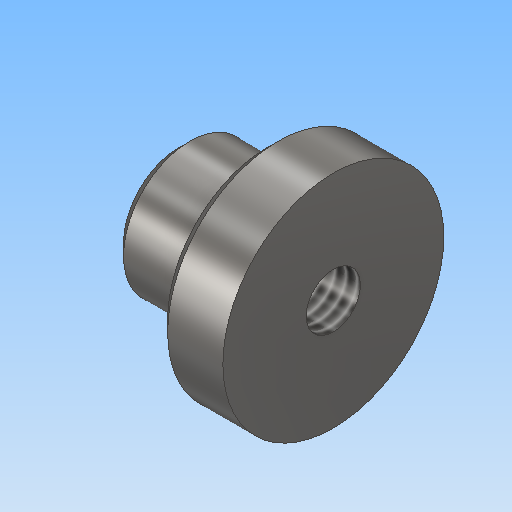
# Autodesk Inventor part: Top_Shaft 1
Saved by Autodesk Inventor 2018.1 (Build 221171000, 171)
## iProperties
Created: 2019-03-18
Part Number: Top_Shaft 1
Material: Stainless Steel
Document SubType Name: Modeling
Designer: James
Density: 8 g/cm^3
Appearance: Semi-Polished
Mass: 2.47594 g
Surface Area: 3.55126 cm^2
Volume: 0.309493 cm^3
Author: James
Autodesk Inventor part; units mm, degrees
ref_plane "YZ Plane" through (0, 0, 0) normal (1, 0, 0) x (0, 1, 0)
ref_plane "XZ Plane" through (0, 0, 0) normal (0, 1, 0) x (-1, 0, 0)
ref_plane "XY Plane" through (0, 0, 0) normal (0, 0, 1) x (1, 0, 0)
sketch "Sketch1" plane through (0, 0, 0) normal (0, 0, 1) x (1, 0, 0)
  line L0 (0, 0) -> (4, 0)
  line L1 (4, 0) -> (4, 3)
  line L2 (4, 3) -> (0, 3)
  line L3 (0, 3) -> (0, 0)
  line L4 (4, 0) -> (7, 0)
  line L5 (7, 0) -> (7, 5)
  line L6 (7, 5) -> (4, 5)
  line L7 (4, 5) -> (4, 0)
  dimension "d0" = 4
  dimension "d1" = 3
  dimension "d2" = 3
  dimension "d3" = 5
  constraints: 16 end point, 4 parallel, 2 horizontal, 2 perpendicular
  measures "d0" distance of L1.end L2.end
  measures "d1" distance of L5.end L6.end
  measures "d2" distance of L2.end L0.start
  measures "d3" distance of L4.end L5.end
revolve "Revolution1" add sketch "Sketch1" angle 360 about axis through (0, 0, 0) along (1, 0, 0)
fillet "Fillet1" radius 0.1 1 edges at (4, -3, 0)
chamfer "Chamfer1" distance 0.5 angle 45 2 edges at (4, -5, 0) (0, -3, 0)
sketch "Sketch2" plane through (0, 0, 0) normal (-1, 0, 0) x (0, 0, 1)
  point P0 (0, 0)
  point P1 (0, 0)
  constraints: 1 coincident
hole "Hole1" at (0, 0, 0) direction (1, 0, 0) diameter 2.459 end through all thread size "M3x0.5" class "6H" standard "ANSI Metric M Profile"
body "Solid1"
